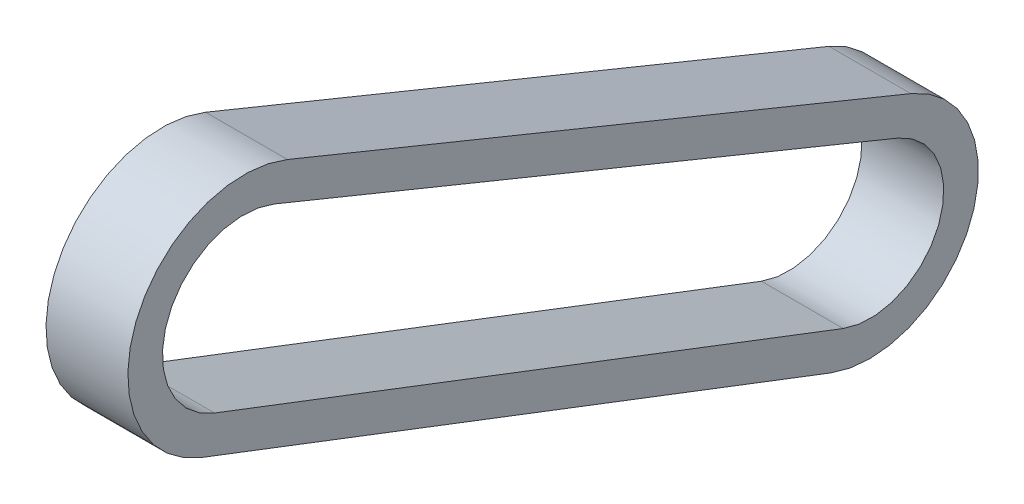
# Autodesk Inventor part: 45tooth belt
Saved by Autodesk Inventor 2023 (Build 270158000, 158)
## iProperties
Created: 2022-09-06
Part Number: 45tooth belt
Material: Generic
Document SubType Name: Modeling
Designer: deli
Density: 1 g/cm^3
Appearance: Default
Author: deli
Autodesk Inventor part; units mm, degrees
ref_plane "YZ Plane" through (0, 0, 0) normal (1, 0, 0) x (0, 1, 0)
ref_plane "XZ Plane" through (0, 0, 0) normal (0, 1, 0) x (-1, 0, 0)
ref_plane "XY Plane" through (0, 0, 0) normal (0, 0, 1) x (1, 0, 0)
sketch "Sketch1" plane through (0, 0, 0) normal (1, 0, 0) x (0, 1, 0)
  circle A0 centre (-294.5036, -350.9294) radius 2 construction
  circle A1 centre (-267.2536, -282.1084) radius 7 construction
  arc A2 (-305.6485, -346.6545) -> (-283.4532, -355.4429) centre (-294.5036, -350.9294) ccw
  arc A3 (-255.4665, -286.9228) -> (-279.1415, -277.5486) centre (-267.2536, -282.1084) ccw
  line L0 (-283.4532, -355.4429) -> (-255.4665, -286.9228)
  line L1 (-279.1415, -277.5486) -> (-305.6485, -346.6545)
  line L2 (-258.9844, -285.486) -> (-286.9711, -354.006)
  arc A4 (-302.1005, -348.0154) -> (-286.9711, -354.006) centre (-294.5036, -350.9294) ccw
  line L3 (-302.1005, -348.0154) -> (-275.5935, -278.9095)
  arc A5 (-258.9844, -285.486) -> (-275.5935, -278.9095) centre (-267.2536, -282.1084) ccw
  point P0 (0, 0)
  dimension "d0" = 23.8732
  dimension "d1" = 25.4648
  dimension "d2" = 3.8
  constraints: 8 end point, 8 point on circle, 4 centre point, 4 tangent, 2 coincident, 3 other
  measures "d0" diameter of A2
  measures "d1" diameter of A3
  measures "d2" distance between parallel lines of L0 L2
extrude "Extrusion1" add sketch "Sketch1" along normal blind 9
body "Solid1"
